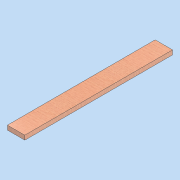
# Autodesk Inventor part: bodyTopPlate
Saved by Autodesk Inventor 2021 (Build 250183000, 183)
## iProperties
Created: 2021-02-01
Part Number: bodyTopPlate
Material: Generic
Document SubType Name: Modeling
Designer: garre
Density: 1 g/cm^3
Appearance: Default
Author: garre
Autodesk Inventor part; units mm, degrees
ref_plane "YZ Plane" through (0, 0, 0) normal (1, 0, 0) x (0, 1, 0)
ref_plane "XZ Plane" through (0, 0, 0) normal (0, 1, 0) x (-1, 0, 0)
ref_plane "XY Plane" through (0, 0, 0) normal (0, 0, 1) x (1, 0, 0)
sketch "Sketch1" plane through (0, 0, 0) normal (0, 1, 0) x (-1, 0, 0)
  line L0 (0, 0) -> (76.2, 0)
  line L1 (76.2, 0) -> (76.2, -647.7)
  line L2 (76.2, -647.7) -> (0, -647.7)
  line L3 (0, -647.7) -> (0, 0)
  dimension "d1" = 76.2
  dimension "d2" = 647.7
  constraints: 8 end point, 2 parallel, 1 horizontal, 1 perpendicular
  measures "d1" distance of L0.start L0.end
  measures "d2" distance of L0.end L1.end
extrude "Extrusion1" add sketch "Sketch1" along normal blind 19.05
equation "\"d1\" = topPlateWidth"
equation "\"d2\" = topPlateLength"
equation "\"d3\" = woodThickness"
equation "\"topPlateLength\" = 647.7"
equation "\"woodThickness\" = 19.05"
equation "\"topPlateWidth\" = 76.2"
body "Solid1"
